Autodesk Fusion 360 part; units mm, degrees
(part 2 of 4)
  line L1019 (-48.5, -47.866) -> (-48, -48.7321)
  line L1020 (-40.5, -47.866) -> (-41, -47)
  line L1021 (-48.5, -41.866) -> (-48, -42.7321)
  line L1022 (-35, -36.7321) -> (-34.5, -35.866)
  line L1023 (-46.5, -41.866) -> (-47, -41)
  line L1024 (-39, -36.7321) -> (-38, -36.7321)
  line L1025 (-45, -42.7321) -> (-44, -42.7321)
  line L1026 (-47, -44) -> (-48, -44)
  line L1027 (-44, -47) -> (-45, -47)
  line L1028 (-48, -48.7321) -> (-47, -48.7321)
  line L1029 (-48, -44) -> (-48.5, -44.866)
  line L1030 (-35, -38) -> (-36, -38)
  line L1031 (-48, -41) -> (-48.5, -41.866)
  line L1032 (-45, -47) -> (-45.5, -47.866)
  line L1033 (-44, -41) -> (-45, -41)
  line L1034 (-38, -38) -> (-39, -38)
  line L1035 (-39, -39.7321) -> (-38, -39.7321)
  line L1036 (-45, -48.7321) -> (-44, -48.7321)
  line L1037 (-45, -41) -> (-45.5, -41.866)
  line L1038 (-42.5, -56.866) -> (-42, -57.7321)
  line L1039 (-40.5, -56.866) -> (-41, -56)
  line L1040 (-44, -54.7321) -> (-43.5, -53.866)
  line L1041 (-42, -51.7321) -> (-41, -51.7321)
  line L1042 (-41, -51.7321) -> (-40.5, -50.866)
  line L1043 (-44, -57.7321) -> (-43.5, -56.866)
  line L1044 (-38, -48.7321) -> (-37.5, -47.866)
  line L1045 (-40.5, -50.866) -> (-41, -50)
  line L1046 (-42, -57.7321) -> (-41, -57.7321)
  line L1047 (-36, -47) -> (-36.5, -47.866)
  line L1048 (-39.5, -47.866) -> (-39, -48.7321)
  line L1049 (-40.5, -53.866) -> (-41, -53)
  line L1050 (-39, -48.7321) -> (-38, -48.7321)
  line L1051 (-42.5, -53.866) -> (-42, -54.7321)
  line L1052 (-41, -57.7321) -> (-40.5, -56.866)
  line L1053 (-41, -50) -> (-42, -50)
  line L1054 (-45.5, -47.866) -> (-45, -48.7321)
  line L1055 (-42, -53) -> (-42.5, -53.866)
  line L1056 (-44, -51.7321) -> (-43.5, -50.866)
  line L1057 (-42, -50) -> (-42.5, -50.866)
  line L1058 (-36.5, -35.866) -> (-36, -36.7321)
  line L1059 (-45.5, -41.866) -> (-45, -42.7321)
  line L1060 (-42, -54.7321) -> (-41, -54.7321)
  line L1061 (-35, -39.7321) -> (-34.5, -38.866)
  line L1062 (-47, -42.7321) -> (-46.5, -41.866)
  line L1063 (-43.5, -53.866) -> (-44, -53)
  line L1064 (-38, -39.7321) -> (-37.5, -38.866)
  line L1065 (-42.5, -50.866) -> (-42, -51.7321)
  line L1066 (-43.5, -50.866) -> (-44, -50)
  line L1067 (-37.5, -38.866) -> (-38, -38)
  line L1068 (-36, -36.7321) -> (-35, -36.7321)
  line L1069 (-36, -39.7321) -> (-35, -39.7321)
  line L1070 (-45.5, -44.866) -> (-45, -45.7321)
  line L1071 (-38, -35) -> (-39, -35)
  line L1072 (-39.5, -38.866) -> (-39, -39.7321)
  line L1073 (-41, -54.7321) -> (-40.5, -53.866)
  line L1074 (-43.5, -56.866) -> (-44, -56)
  line L1075 (-42, -56) -> (-42.5, -56.866)
  line L1076 (-39.5, -35.866) -> (-39, -36.7321)
  line L1077 (-35, -35) -> (-36, -35)
  line L1078 (-41, -56) -> (-42, -56)
  line L1079 (-48, -47) -> (-48.5, -47.866)
  line L1080 (-39, -38) -> (-39.5, -38.866)
  line L1081 (-34.5, -38.866) -> (-35, -38)
  line L1082 (-41, -53) -> (-42, -53)
  line L1083 (-47, -48.7321) -> (-46.5, -47.866)
  line L1084 (-36, -35) -> (-36.5, -35.866)
  line L1085 (-46.5, -47.866) -> (-47, -47)
  line L1086 (-38, -36.7321) -> (-37.5, -35.866)
  line L1087 (-36, -38) -> (-36.5, -38.866)
  line L1088 (-36.5, -38.866) -> (-36, -39.7321)
  line L1089 (-48, -42.7321) -> (-47, -42.7321)
  line L1090 (-46.5, -44.866) -> (-47, -44)
  line L1091 (-34.5, -35.866) -> (-35, -35)
  line L1092 (-59, -54.7321) -> (-58.5, -53.866)
  line L1093 (-57, -47) -> (-57.5, -47.866)
  line L1094 (-60, -51.7321) -> (-59, -51.7321)
  line L1095 (-56, -47) -> (-57, -47)
  line L1096 (-60, -57.7321) -> (-59, -57.7321)
  line L1097 (-58.5, -56.866) -> (-59, -56)
  line L1098 (-53, -54.7321) -> (-52.5, -53.866)
  line L1099 (-52.5, -50.866) -> (-53, -50)
  line L1100 (-51, -56) -> (-51.5, -56.866)
  line L1101 (-50, -50) -> (-51, -50)
  line L1102 (-63, -54.7321) -> (-62, -54.7321)
  line L1103 (-59, -51.7321) -> (-58.5, -50.866)
  line L1104 (-53, -57.7321) -> (-52.5, -56.866)
  line L1105 (-50, -53) -> (-51, -53)
  line L1106 (-60, -54.7321) -> (-59, -54.7321)
  line L1107 (-54, -47) -> (-54.5, -47.866)
  line L1108 (-63.5, -56.866) -> (-63, -57.7321)
  line L1109 (-55.5, -47.866) -> (-56, -47)
  line L1110 (-57, -48.7321) -> (-56, -48.7321)
  line L1111 (-54.5, -44.866) -> (-54, -45.7321)
  line L1112 (-63, -53) -> (-63.5, -53.866)
  line L1113 (-62, -54.7321) -> (-61.5, -53.866)
  line L1114 (-51, -57.7321) -> (-50, -57.7321)
  line L1115 (-57, -41) -> (-57.5, -41.866)
  line L1116 (-60.5, -53.866) -> (-60, -54.7321)
  line L1117 (-57.5, -41.866) -> (-57, -42.7321)
  line L1118 (-63.5, -50.866) -> (-63, -51.7321)
  line L1119 (-60, -53) -> (-60.5, -53.866)
  line L1120 (-59, -50) -> (-60, -50)
  line L1121 (-56, -41) -> (-57, -41)
  line L1122 (-52.5, -53.866) -> (-53, -53)
  line L1123 (-63, -56) -> (-63.5, -56.866)
  line L1124 (-62, -56) -> (-63, -56)
  line L1125 (-60, -56) -> (-60.5, -56.866)
  line L1126 (-49.5, -50.866) -> (-50, -50)
  line L1127 (-62, -50) -> (-63, -50)
  line L1128 (-61.5, -53.866) -> (-62, -53)
  line L1129 (-60.5, -56.866) -> (-60, -57.7321)
  line L1130 (-62, -57.7321) -> (-61.5, -56.866)
  line L1131 (-59, -57.7321) -> (-58.5, -56.866)
  line L1132 (-61.5, -56.866) -> (-62, -56)
  line L1133 (-62, -51.7321) -> (-61.5, -50.866)
  line L1134 (-63, -50) -> (-63.5, -50.866)
  line L1135 (-58.5, -50.866) -> (-59, -50)
  line L1136 (-60, -50) -> (-60.5, -50.866)
  line L1137 (-57, -44) -> (-57.5, -44.866)
  line L1138 (-50, -51.7321) -> (-49.5, -50.866)
  line L1139 (-51, -47) -> (-51.5, -47.866)
  line L1140 (-51, -48.7321) -> (-50, -48.7321)
  line L1141 (-35, -54.7321) -> (-34.5, -53.866)
  line L1142 (-53, -48.7321) -> (-52.5, -47.866)
  line L1143 (-60.5, -38.866) -> (-60, -39.7321)
  line L1144 (-60, -36.7321) -> (-59, -36.7321)
  line L1145 (-38, -54.7321) -> (-37.5, -53.866)
  line L1146 (-52.5, -41.866) -> (-53, -41)
  line L1147 (-36.5, -53.866) -> (-36, -54.7321)
  line L1148 (-62, -38) -> (-63, -38)
  line L1149 (-58.5, -35.866) -> (-59, -35)
  line L1150 (-39, -53) -> (-39.5, -53.866)
  line L1151 (-51, -42.7321) -> (-50, -42.7321)
  line L1152 (-52.5, -47.866) -> (-53, -47)
  line L1153 (-53, -45.7321) -> (-52.5, -44.866)
  line L1154 (-60, -35) -> (-60.5, -35.866)
  line L1155 (-38, -50) -> (-39, -50)
  line L1156 (-50, -42.7321) -> (-49.5, -41.866)
  line L1157 (-63, -39.7321) -> (-62, -39.7321)
  line L1158 (-59, -35) -> (-60, -35)
  line L1159 (-63.5, -35.866) -> (-63, -36.7321)
  line L1160 (-63, -38) -> (-63.5, -38.866)
  line L1161 (-61.5, -35.866) -> (-62, -35)
  line L1162 (-60, -39.7321) -> (-59, -39.7321)
  line L1163 (-60.5, -35.866) -> (-60, -36.7321)
  line L1164 (-62, -36.7321) -> (-61.5, -35.866)
  line L1165 (-62, -39.7321) -> (-61.5, -38.866)
  line L1166 (-61.5, -38.866) -> (-62, -38)
  line L1167 (-51, -41) -> (-51.5, -41.866)
  line L1168 (-36, -56) -> (-36.5, -56.866)
  line L1169 (-51.5, -44.866) -> (-51, -45.7321)
  line L1170 (-36, -57.7321) -> (-35, -57.7321)
  line L1171 (-36, -53) -> (-36.5, -53.866)
  line L1172 (-34.5, -50.866) -> (-35, -50)
  line L1173 (-49.5, -41.866) -> (-50, -41)
  line L1174 (-35, -57.7321) -> (-34.5, -56.866)
  line L1175 (-37.5, -53.866) -> (-38, -53)
  line L1176 (-34.5, -56.866) -> (-35, -56)
  line L1177 (-37.5, -50.866) -> (-38, -50)
  line L1178 (-39, -54.7321) -> (-38, -54.7321)
  line L1179 (-38, -51.7321) -> (-37.5, -50.866)
  line L1180 (-36, -51.7321) -> (-35, -51.7321)
  line L1181 (-39.5, -53.866) -> (-39, -54.7321)
  line L1182 (-51.5, -41.866) -> (-51, -42.7321)
  line L1183 (-39.5, -56.866) -> (-39, -57.7321)
  line L1184 (-49.5, -44.866) -> (-50, -44)
  line L1185 (-50, -45.7321) -> (-49.5, -44.866)
  line L1186 (-57, -39.7321) -> (-56, -39.7321)
  line L1187 (-37.5, -56.866) -> (-38, -56)
  line L1188 (-38, -56) -> (-39, -56)
  line L1189 (-34.5, -53.866) -> (-35, -53)
  line L1190 (-36, -54.7321) -> (-35, -54.7321)
  line L1191 (-64.5, -56.866) -> (-65, -56)
  line L1192 (-64.5, -41.866) -> (-65, -41)
  line L1193 (-69.5, -50.866) -> (-69, -51.7321)
  line L1194 (-65, -42.7321) -> (-64.5, -41.866)
  line L1195 (-64.5, -44.866) -> (-65, -44)
  line L1196 (-66, -42.7321) -> (-65, -42.7321)
  line L1197 (-68, -50) -> (-69, -50)
  line L1198 (-66.5, -41.866) -> (-66, -42.7321)
  line L1199 (-69, -47) -> (-69.5, -47.866)
  line L1200 (-68, -51.7321) -> (-67.5, -50.866)
  line L1201 (-69, -56) -> (-69.5, -56.866)
  line L1202 (-66.5, -44.866) -> (-66, -45.7321)
  line L1203 (-68, -53) -> (-69, -53)
  line L1204 (-69, -51.7321) -> (-68, -51.7321)
  line L1205 (-67.5, -44.866) -> (-68, -44)
  line L1206 (-69, -53) -> (-69.5, -53.866)
  line L1207 (-66, -50) -> (-66.5, -50.866)
  line L1208 (-69, -57.7321) -> (-68, -57.7321)
  line L1209 (-66.5, -47.866) -> (-66, -48.7321)
  line L1210 (-68, -45.7321) -> (-67.5, -44.866)
  line L1211 (-66, -45.7321) -> (-65, -45.7321)
  line L1212 (-69.5, -56.866) -> (-69, -57.7321)
  line L1213 (-68, -42.7321) -> (-67.5, -41.866)
  line L1214 (-69, -42.7321) -> (-68, -42.7321)
  line L1215 (-69.5, -44.866) -> (-69, -45.7321)
  line L1216 (-66.5, -50.866) -> (-66, -51.7321)
  line L1217 (-69, -45.7321) -> (-68, -45.7321)
  line L1218 (-68, -48.7321) -> (-67.5, -47.866)
  line L1219 (-65, -44) -> (-66, -44)
  line L1220 (-11, -51.7321) -> (-10.5, -50.866)
  line L1221 (-21, -38) -> (-21.5, -38.866)
  line L1222 (-13.5, -38.866) -> (-14, -38)
  line L1223 (-16.5, -35.866) -> (-17, -35)
  line L1224 (-11, -50) -> (-12, -50)
  line L1225 (-12, -57.7321) -> (-11, -57.7321)
  line L1226 (-14, -35) -> (-15, -35)
  line L1227 (-24, -38) -> (-24.5, -38.866)
  line L1228 (-14, -53) -> (-15, -53)
  line L1229 (-18, -38) -> (-18.5, -38.866)
  line L1230 (-10.5, -35.866) -> (-11, -35)
  line L1231 (-17, -36.7321) -> (-16.5, -35.866)
  line L1232 (-11, -53) -> (-12, -53)
  line L1233 (-24.5, -35.866) -> (-24, -36.7321)
  line L1234 (-20, -35) -> (-21, -35)
  line L1235 (-12, -38) -> (-12.5, -38.866)
  line L1236 (-17, -39.7321) -> (-16.5, -38.866)
  line L1237 (-15.5, -50.866) -> (-15, -51.7321)
  line L1238 (-25.5, -35.866) -> (-26, -35)
  line L1239 (-18, -57.7321) -> (-17, -57.7321)
  line L1240 (-24, -36.7321) -> (-23, -36.7321)
  line L1241 (-12, -35) -> (-12.5, -35.866)
  line L1242 (-23, -39.7321) -> (-22.5, -38.866)
  line L1243 (-17, -38) -> (-18, -38)
  line L1244 (-21, -36.7321) -> (-20, -36.7321)
  line L1245 (-24, -39.7321) -> (-23, -39.7321)
  line L1246 (-12.5, -53.866) -> (-12, -54.7321)
  line L1247 (-18.5, -50.866) -> (-18, -51.7321)
  line L1248 (-14, -54.7321) -> (-13.5, -53.866)
  line L1249 (-14, -38) -> (-15, -38)
  line L1250 (-10.5, -38.866) -> (-11, -38)
  line L1251 (-24, -35) -> (-24.5, -35.866)
  line L1252 (-27, -35) -> (-27.5, -35.866)
  line L1253 (-22.5, -35.866) -> (-23, -35)
  line L1254 (-12, -36.7321) -> (-11, -36.7321)
  line L1255 (-22.5, -38.866) -> (-23, -38)
  line L1256 (-23, -38) -> (-24, -38)
  line L1257 (-14, -50) -> (-15, -50)
  line L1258 (-19.5, -35.866) -> (-20, -35)
  line L1259 (-11, -38) -> (-12, -38)
  line L1260 (-19.5, -38.866) -> (-20, -38)
  line L1261 (-11, -39.7321) -> (-10.5, -38.866)
  line L1262 (-12.5, -50.866) -> (-12, -51.7321)
  line L1263 (-15, -36.7321) -> (-14, -36.7321)
  line L1264 (-27.5, -38.866) -> (-27, -39.7321)
  line L1265 (-15, -35) -> (-15.5, -35.866)
  line L1266 (-12.5, -38.866) -> (-12, -39.7321)
  line L1267 (-27.5, -35.866) -> (-27, -36.7321)
  line L1268 (-14, -51.7321) -> (-13.5, -50.866)
  line L1269 (-21.5, -38.866) -> (-21, -39.7321)
  line L1270 (-11, -36.7321) -> (-10.5, -35.866)
  line L1271 (-27, -39.7321) -> (-26, -39.7321)
  line L1272 (-20, -38) -> (-21, -38)
  line L1273 (-11, -57.7321) -> (-10.5, -56.866)
  line L1274 (-12, -53) -> (-12.5, -53.866)
  line L1275 (-10.5, -50.866) -> (-11, -50)
  line L1276 (-12, -39.7321) -> (-11, -39.7321)
  line L1277 (-14, -57.7321) -> (-13.5, -56.866)
  line L1278 (-26, -39.7321) -> (-25.5, -38.866)
  line L1279 (-15, -39.7321) -> (-14, -39.7321)
  line L1280 (-15.5, -38.866) -> (-15, -39.7321)
  line L1281 (-18, -36.7321) -> (-17, -36.7321)
  line L1282 (-12.5, -56.866) -> (-12, -57.7321)
  line L1283 (-20, -36.7321) -> (-19.5, -35.866)
  line L1284 (-13.5, -56.866) -> (-14, -56)
  line L1285 (-24.5, -38.866) -> (-24, -39.7321)
  line L1286 (-18, -39.7321) -> (-17, -39.7321)
  line L1287 (-12, -54.7321) -> (-11, -54.7321)
  line L1288 (-10.5, -56.866) -> (-11, -56)
  line L1289 (-14, -36.7321) -> (-13.5, -35.866)
  line L1290 (-10.5, -53.866) -> (-11, -53)
  line L1291 (-21.5, -35.866) -> (-21, -36.7321)
  line L1292 (-12.5, -35.866) -> (-12, -36.7321)
  line L1293 (-21, -39.7321) -> (-20, -39.7321)
  line L1294 (-14, -39.7321) -> (-13.5, -38.866)
  line L1295 (-12, -50) -> (-12.5, -50.866)
  line L1296 (-12, -51.7321) -> (-11, -51.7321)
  line L1297 (-26, -36.7321) -> (-25.5, -35.866)
  line L1298 (-18, -35) -> (-18.5, -35.866)
  line L1299 (-27, -38) -> (-27.5, -38.866)
  line L1300 (-13.5, -35.866) -> (-14, -35)
  line L1301 (-23, -42.7321) -> (-22.5, -41.866)
  line L1302 (-22.5, -44.866) -> (-23, -44)
  line L1303 (-21, -45.7321) -> (-20, -45.7321)
  line L1304 (-20, -44) -> (-21, -44)
  line L1305 (-25.5, -38.866) -> (-26, -38)
  line L1306 (-26, -38) -> (-27, -38)
  line L1307 (-22.5, -47.866) -> (-23, -47)
  line L1308 (-17, -51.7321) -> (-16.5, -50.866)
  line L1309 (-17, -50) -> (-18, -50)
  line L1310 (-15, -53) -> (-15.5, -53.866)
  line L1311 (-16.5, -38.866) -> (-17, -38)
  line L1312 (-16.5, -53.866) -> (-17, -53)
  line L1313 (-14, -56) -> (-15, -56)
  line L1314 (-20, -39.7321) -> (-19.5, -38.866)
  line L1315 (-18, -50) -> (-18.5, -50.866)
  line L1316 (-21, -35) -> (-21.5, -35.866)
  line L1317 (-18.5, -38.866) -> (-18, -39.7321)
  line L1318 (-17, -56) -> (-18, -56)
  line L1319 (-20, -41) -> (-21, -41)
  line L1320 (-15, -50) -> (-15.5, -50.866)
  line L1321 (-15.5, -53.866) -> (-15, -54.7321)
  line L1322 (-17, -53) -> (-18, -53)
  line L1323 (-18.5, -53.866) -> (-18, -54.7321)
  line L1324 (-19.5, -41.866) -> (-20, -41)
  line L1325 (-15, -54.7321) -> (-14, -54.7321)
  line L1326 (-16.5, -50.866) -> (-17, -50)
  line L1327 (-22.5, -41.866) -> (-23, -41)
  line L1328 (-19.5, -47.866) -> (-20, -47)
  line L1329 (-18, -51.7321) -> (-17, -51.7321)
  line L1330 (-18, -53) -> (-18.5, -53.866)
  line L1331 (-18, -54.7321) -> (-17, -54.7321)
  line L1332 (-17, -57.7321) -> (-16.5, -56.866)
  line L1333 (-21, -42.7321) -> (-20, -42.7321)
  line L1334 (-20, -47) -> (-21, -47)
  line L1335 (-17, -54.7321) -> (-16.5, -53.866)
  line L1336 (-15, -51.7321) -> (-14, -51.7321)
  line L1337 (-23, -48.7321) -> (-22.5, -47.866)
  line L1338 (-15.5, -56.866) -> (-15, -57.7321)
  line L1339 (-21.5, -41.866) -> (-21, -42.7321)
  line L1340 (-20, -45.7321) -> (-19.5, -44.866)
  line L1341 (-15, -56) -> (-15.5, -56.866)
  line L1342 (-18, -56) -> (-18.5, -56.866)
  line L1343 (-15, -57.7321) -> (-14, -57.7321)
  line L1344 (-19.5, -44.866) -> (-20, -44)
  line L1345 (-29, -39.7321) -> (-28.5, -38.866)
  line L1346 (-16.5, -56.866) -> (-17, -56)
  line L1347 (-18.5, -56.866) -> (-18, -57.7321)
  line L1348 (-21, -41) -> (-21.5, -41.866)
  line L1349 (-23, -47) -> (-24, -47)
  line L1350 (-26, -41) -> (-27, -41)
  line L1351 (-32, -36.7321) -> (-31.5, -35.866)
  line L1352 (-21.5, -47.866) -> (-21, -48.7321)
  line L1353 (-24, -42.7321) -> (-23, -42.7321)
  line L1354 (-26, -42.7321) -> (-25.5, -41.866)
  line L1355 (-27, -42.7321) -> (-26, -42.7321)
  line L1356 (-29, -38) -> (-30, -38)
  line L1357 (-27, -48.7321) -> (-26, -48.7321)
  line L1358 (-33.5, -35.866) -> (-33, -36.7321)
  line L1359 (-24.5, -44.866) -> (-24, -45.7321)
  line L1360 (-21, -47) -> (-21.5, -47.866)
  line L1361 (-20, -48.7321) -> (-19.5, -47.866)
  line L1362 (-23, -44) -> (-24, -44)
  line L1363 (-27.5, -41.866) -> (-27, -42.7321)
  line L1364 (-24.5, -47.866) -> (-24, -48.7321)
  line L1365 (-31.5, -35.866) -> (-32, -35)
  line L1366 (-23, -45.7321) -> (-22.5, -44.866)
  line L1367 (-21.5, -44.866) -> (-21, -45.7321)
  line L1368 (-24, -45.7321) -> (-23, -45.7321)
  line L1369 (-28.5, -38.866) -> (-29, -38)
  line L1370 (-33.5, -38.866) -> (-33, -39.7321)
  line L1371 (-21, -48.7321) -> (-20, -48.7321)
  line L1372 (-21, -44) -> (-21.5, -44.866)
  line L1373 (-20, -42.7321) -> (-19.5, -41.866)
  line L1374 (-26, -45.7321) -> (-25.5, -44.866)
  line L1375 (-29, -36.7321) -> (-28.5, -35.866)
  line L1376 (-27.5, -44.866) -> (-27, -45.7321)
  line L1377 (-29, -51.7321) -> (-28.5, -50.866)
  line L1378 (-44, -35) -> (-45, -35)
  line L1379 (-28.5, -50.866) -> (-29, -50)
  line L1380 (-41, -39.7321) -> (-40.5, -38.866)
  line L1381 (-31.5, -56.866) -> (-32, -56)
  line L1382 (-45, -36.7321) -> (-44, -36.7321)
  line L1383 (-43.5, -35.866) -> (-44, -35)
  line L1384 (-44, -36.7321) -> (-43.5, -35.866)
  line L1385 (-48, -39.7321) -> (-47, -39.7321)
  line L1386 (-32, -54.7321) -> (-31.5, -53.866)
  line L1387 (-43.5, -38.866) -> (-44, -38)
  line L1388 (-42, -35) -> (-42.5, -35.866)
  line L1389 (-42.5, -35.866) -> (-42, -36.7321)
  line L1390 (-28.5, -56.866) -> (-29, -56)
  line L1391 (-31.5, -53.866) -> (-32, -53)
  line L1392 (-42.5, -38.866) -> (-42, -39.7321)
  line L1393 (-33, -53) -> (-33.5, -53.866)
  line L1394 (-29, -54.7321) -> (-28.5, -53.866)
  line L1395 (-33.5, -53.866) -> (-33, -54.7321)
  line L1396 (-28.5, -53.866) -> (-29, -53)
  line L1397 (-45.5, -38.866) -> (-45, -39.7321)
  line L1398 (-47, -39.7321) -> (-46.5, -38.866)
  line L1399 (-40.5, -41.866) -> (-41, -41)
  line L1400 (-30.5, -50.866) -> (-30, -51.7321)
  line L1401 (-42, -38) -> (-42.5, -38.866)
  line L1402 (-29, -56) -> (-30, -56)
  line L1403 (-33, -50) -> (-33.5, -50.866)
  line L1404 (-33, -54.7321) -> (-32, -54.7321)
  line L1405 (-33, -57.7321) -> (-32, -57.7321)
  line L1406 (-48.5, -38.866) -> (-48, -39.7321)
  line L1407 (-40.5, -38.866) -> (-41, -38)
  line L1408 (-45, -38) -> (-45.5, -38.866)
  line L1409 (-44, -38) -> (-45, -38)
  line L1410 (-32, -56) -> (-33, -56)
  line L1411 (-32, -51.7321) -> (-31.5, -50.866)
  line L1412 (-41, -38) -> (-42, -38)
  line L1413 (-45, -35) -> (-45.5, -35.866)
  line L1414 (-30, -50) -> (-30.5, -50.866)
  line L1415 (-41, -35) -> (-42, -35)
  line L1416 (-32, -53) -> (-33, -53)
  line L1417 (-51.5, -35.866) -> (-51, -36.7321)
  line L1418 (-57.5, -38.866) -> (-57, -39.7321)
  line L1419 (-53, -36.7321) -> (-52.5, -35.866)
  line L1420 (-51.5, -38.866) -> (-51, -39.7321)
  line L1421 (-39, -51.7321) -> (-38, -51.7321)
  line L1422 (-54, -35) -> (-54.5, -35.866)
  line L1423 (-56, -35) -> (-57, -35)
  line L1424 (-54, -39.7321) -> (-53, -39.7321)
  line L1425 (-53, -38) -> (-54, -38)
  line L1426 (-39, -50) -> (-39.5, -50.866)
  line L1427 (-57, -38) -> (-57.5, -38.866)
  line L1428 (-35, -51.7321) -> (-34.5, -50.866)
  line L1429 (-50, -39.7321) -> (-49.5, -38.866)
  line L1430 (-50, -38) -> (-51, -38)
  line L1431 (-21, -57.7321) -> (-20, -57.7321)
  line L1432 (-30, -39.7321) -> (-29, -39.7321)
  line L1433 (-21.5, -53.866) -> (-21, -54.7321)
  line L1434 (-32, -39.7321) -> (-31.5, -38.866)
  line L1435 (-24, -41) -> (-24.5, -41.866)
  line L1436 (-33, -36.7321) -> (-32, -36.7321)
  line L1437 (-27, -47) -> (-27.5, -47.866)
  line L1438 (-23, -41) -> (-24, -41)
  line L1439 (-33, -39.7321) -> (-32, -39.7321)
  line L1440 (-30, -38) -> (-30.5, -38.866)
  line L1441 (-25.5, -44.866) -> (-26, -44)
  line L1442 (-23, -51.7321) -> (-22.5, -50.866)
  line L1443 (-30, -36.7321) -> (-29, -36.7321)
  line L1444 (-25.5, -41.866) -> (-26, -41)
  line L1445 (-32, -38) -> (-33, -38)
  line L1446 (-21, -56) -> (-21.5, -56.866)
  line L1447 (-32, -35) -> (-33, -35)
  line L1448 (-29, -35) -> (-30, -35)
  line L1449 (-21, -51.7321) -> (-20, -51.7321)
  line L1450 (-24, -47) -> (-24.5, -47.866)
  line L1451 (-24, -44) -> (-24.5, -44.866)
  line L1452 (-30.5, -35.866) -> (-30, -36.7321)
  line L1453 (-33, -38) -> (-33.5, -38.866)
  line L1454 (-31.5, -38.866) -> (-32, -38)
  line L1455 (-24.5, -41.866) -> (-24, -42.7321)
  line L1456 (-27, -45.7321) -> (-26, -45.7321)
  line L1457 (-30, -35) -> (-30.5, -35.866)
  line L1458 (-27.5, -47.866) -> (-27, -48.7321)
  line L1459 (-28.5, -35.866) -> (-29, -35)
  line L1460 (-26, -48.7321) -> (-25.5, -47.866)
  line L1461 (-25.5, -47.866) -> (-26, -47)
  line L1462 (-24, -48.7321) -> (-23, -48.7321)
  line L1463 (-30.5, -38.866) -> (-30, -39.7321)
  line L1464 (-27, -44) -> (-27.5, -44.866)
  line L1465 (-26, -44) -> (-27, -44)
  line L1466 (-27, -41) -> (-27.5, -41.866)
  line L1467 (-33, -35) -> (-33.5, -35.866)
  line L1468 (-26, -47) -> (-27, -47)
  line L1469 (-32, -47) -> (-33, -47)
  line L1470 (-29, -47) -> (-30, -47)
  line L1471 (-33.5, -41.866) -> (-33, -42.7321)
  line L1472 (-30.5, -41.866) -> (-30, -42.7321)
  line L1473 (-22.5, -53.866) -> (-23, -53)
  line L1474 (-21, -50) -> (-21.5, -50.866)
  line L1475 (-30, -47) -> (-30.5, -47.866)
  line L1476 (-21.5, -50.866) -> (-21, -51.7321)
  line L1477 (-21.5, -56.866) -> (-21, -57.7321)
  line L1478 (-20, -50) -> (-21, -50)
  line L1479 (-20, -53) -> (-21, -53)
  line L1480 (-33, -44) -> (-33.5, -44.866)
  line L1481 (-31.5, -41.866) -> (-32, -41)
  line L1482 (-31.5, -47.866) -> (-32, -47)
  line L1483 (-20, -51.7321) -> (-19.5, -50.866)
  line L1484 (-20, -56) -> (-21, -56)
  line L1485 (-23, -57.7321) -> (-22.5, -56.866)
  line L1486 (-30.5, -47.866) -> (-30, -48.7321)
  line L1487 (-33, -45.7321) -> (-32, -45.7321)
  line L1488 (-21, -54.7321) -> (-20, -54.7321)
  line L1489 (-23, -54.7321) -> (-22.5, -53.866)
  line L1490 (-19.5, -53.866) -> (-20, -53)
  line L1491 (-30, -42.7321) -> (-29, -42.7321)
  line L1492 (-29, -45.7321) -> (-28.5, -44.866)
  line L1493 (-20, -57.7321) -> (-19.5, -56.866)
  line L1494 (-19.5, -50.866) -> (-20, -50)
  line L1495 (-28.5, -47.866) -> (-29, -47)
  line L1496 (-22.5, -50.866) -> (-23, -50)
  line L1497 (-21, -53) -> (-21.5, -53.866)
  line L1498 (-19.5, -56.866) -> (-20, -56)
  line L1499 (-22.5, -56.866) -> (-23, -56)
  line L1500 (-20, -54.7321) -> (-19.5, -53.866)
  line L1501 (-13.5, -41.866) -> (-14, -41)
  line L1502 (-15, -38) -> (-15.5, -38.866)
  line L1503 (-16.5, -44.866) -> (-17, -44)
  line L1504 (-13.5, -50.866) -> (-14, -50)
  line L1505 (-13.5, -44.866) -> (-14, -44)
  line L1506 (-11, -54.7321) -> (-10.5, -53.866)
  line L1507 (-12, -44) -> (-12.5, -44.866)
  line L1508 (-18, -41) -> (-18.5, -41.866)
  line L1509 (-18.5, -35.866) -> (-18, -36.7321)
  line L1510 (-15, -48.7321) -> (-14, -48.7321)
  line L1511 (-10.5, -41.866) -> (-11, -41)
  line L1512 (-11, -42.7321) -> (-10.5, -41.866)
  line L1513 (-12.5, -41.866) -> (-12, -42.7321)
  line L1514 (-11, -47) -> (-12, -47)
  line L1515 (-13.5, -47.866) -> (-14, -47)
  line L1516 (-11, -56) -> (-12, -56)
  line L1517 (-15, -42.7321) -> (-14, -42.7321)
  line L1518 (-17, -48.7321) -> (-16.5, -47.866)
  line L1519 (-16.5, -47.866) -> (-17, -47)
  line L1520 (-17, -45.7321) -> (-16.5, -44.866)
  line L1521 (-11, -48.7321) -> (-10.5, -47.866)
  line L1522 (-27, -36.7321) -> (-26, -36.7321)
  line L1523 (-14, -47) -> (-15, -47)
  line L1524 (-14, -42.7321) -> (-13.5, -41.866)
  line L1525 (-14, -41) -> (-15, -41)
  line L1526 (-11, -35) -> (-12, -35)
  line L1527 (-17, -35) -> (-18, -35)
  line L1528 (-18.5, -47.866) -> (-18, -48.7321)
  line L1529 (-15.5, -44.866) -> (-15, -45.7321)
  line L1530 (-10.5, -44.866) -> (-11, -44)
  line L1531 (-26, -35) -> (-27, -35)
  line L1532 (-13.5, -53.866) -> (-14, -53)
  line L1533 (-17, -41) -> (-18, -41)
  line L1534 (-15.5, -35.866) -> (-15, -36.7321)
  line L1535 (-12, -41) -> (-12.5, -41.866)
  line L1536 (-15, -45.7321) -> (-14, -45.7321)
  line L1537 (-11, -44) -> (-12, -44)
  line L1538 (-14, -45.7321) -> (-13.5, -44.866)
  line L1539 (-23, -36.7321) -> (-22.5, -35.866)
  line L1540 (-23, -35) -> (-24, -35)
  line L1541 (-12, -56) -> (-12.5, -56.866)
  line L1542 (-17, -44) -> (-18, -44)
  line L1543 (-12, -47) -> (-12.5, -47.866)
  line L1544 (-11, -45.7321) -> (-10.5, -44.866)
  line L1545 (-11, -41) -> (-12, -41)
  line L1546 (-18.5, -41.866) -> (-18, -42.7321)
  line L1547 (-12, -45.7321) -> (-11, -45.7321)
  line L1548 (-12, -48.7321) -> (-11, -48.7321)
  line L1549 (-15, -41) -> (-15.5, -41.866)
  line L1550 (-10.5, -47.866) -> (-11, -47)
  line L1551 (-12.5, -44.866) -> (-12, -45.7321)
  line L1552 (-16.5, -41.866) -> (-17, -41)
  line L1553 (-12.5, -47.866) -> (-12, -48.7321)
  line L1554 (-15.5, -41.866) -> (-15, -42.7321)
  line L1555 (-14, -48.7321) -> (-13.5, -47.866)
  line L1556 (-18, -48.7321) -> (-17, -48.7321)
  line L1557 (-18.5, -44.866) -> (-18, -45.7321)
  line L1558 (-15, -44) -> (-15.5, -44.866)
  line L1559 (-17, -47) -> (-18, -47)
  line L1560 (-15, -47) -> (-15.5, -47.866)
  line L1561 (-14, -44) -> (-15, -44)
  line L1562 (-18, -44) -> (-18.5, -44.866)
  line L1563 (-15.5, -47.866) -> (-15, -48.7321)
  line L1564 (-18, -42.7321) -> (-17, -42.7321)
  line L1565 (-17, -42.7321) -> (-16.5, -41.866)
  line L1566 (-12, -42.7321) -> (-11, -42.7321)
  line L1567 (-18, -45.7321) -> (-17, -45.7321)
  line L1568 (-18, -47) -> (-18.5, -47.866)
  line L1569 (-52.5, -44.866) -> (-53, -44)
  line L1570 (-50, -47) -> (-51, -47)
  line L1571 (-61.5, -47.866) -> (-62, -47)
  line L1572 (-60, -42.7321) -> (-59, -42.7321)
  line L1573 (-63, -35) -> (-63.5, -35.866)
  line L1574 (-50, -41) -> (-51, -41)
  line L1575 (-59, -42.7321) -> (-58.5, -41.866)
  line L1576 (-60.5, -44.866) -> (-60, -45.7321)
  line L1577 (-59, -41) -> (-60, -41)
  line L1578 (-60, -48.7321) -> (-59, -48.7321)
  line L1579 (-58.5, -41.866) -> (-59, -41)
  line L1580 (-60, -45.7321) -> (-59, -45.7321)
  line L1581 (-60, -47) -> (-60.5, -47.866)
  line L1582 (-62, -42.7321) -> (-61.5, -41.866)
  line L1583 (-63.5, -41.866) -> (-63, -42.7321)
  line L1584 (-59, -48.7321) -> (-58.5, -47.866)
  line L1585 (-63, -48.7321) -> (-62, -48.7321)
  line L1586 (-59, -39.7321) -> (-58.5, -38.866)
  line L1587 (-63.5, -47.866) -> (-63, -48.7321)
  line L1588 (-59, -45.7321) -> (-58.5, -44.866)
  line L1589 (-58.5, -47.866) -> (-59, -47)
  line L1590 (-51.5, -47.866) -> (-51, -48.7321)
  line L1591 (-62, -47) -> (-63, -47)
  line L1592 (-59, -47) -> (-60, -47)
  line L1593 (-50, -44) -> (-51, -44)
  line L1594 (-61.5, -44.866) -> (-62, -44)
  line L1595 (-51, -45.7321) -> (-50, -45.7321)
  line L1596 (-58.5, -44.866) -> (-59, -44)
  line L1597 (-63, -47) -> (-63.5, -47.866)
  line L1598 (-62, -48.7321) -> (-61.5, -47.866)
  line L1599 (-61.5, -41.866) -> (-62, -41)
  line L1600 (-59, -38) -> (-60, -38)
  line L1601 (-62, -45.7321) -> (-61.5, -44.866)
  line L1602 (-51, -44) -> (-51.5, -44.866)
  line L1603 (-60, -38) -> (-60.5, -38.866)
  line L1604 (-63, -41) -> (-63.5, -41.866)
  line L1605 (-62, -41) -> (-63, -41)
  line L1606 (-63.5, -38.866) -> (-63, -39.7321)
  line L1607 (-49.5, -47.866) -> (-50, -47)
  line L1608 (-53, -42.7321) -> (-52.5, -41.866)
  line L1609 (-50, -48.7321) -> (-49.5, -47.866)
  line L1610 (-62, -35) -> (-63, -35)
  line L1611 (-59, -36.7321) -> (-58.5, -35.866)
  line L1612 (-63, -36.7321) -> (-62, -36.7321)
  line L1613 (-58.5, -38.866) -> (-59, -38)
  line L1614 (-63, -42.7321) -> (-62, -42.7321)
  line L1615 (-61.5, -50.866) -> (-62, -50)
  line L1616 (-54.5, -47.866) -> (-54, -48.7321)
  line L1617 (-63.5, -44.866) -> (-63, -45.7321)
  line L1618 (-56, -45.7321) -> (-55.5, -44.866)
  line L1619 (-60, -44) -> (-60.5, -44.866)
  line L1620 (-63, -44) -> (-63.5, -44.866)
  line L1621 (-54, -42.7321) -> (-53, -42.7321)
  line L1622 (-57, -42.7321) -> (-56, -42.7321)
  line L1623 (-62, -53) -> (-63, -53)
  line L1624 (-58.5, -53.866) -> (-59, -53)
  line L1625 (-59, -53) -> (-60, -53)
  line L1626 (-63, -51.7321) -> (-62, -51.7321)
  line L1627 (-54, -44) -> (-54.5, -44.866)
  line L1628 (-55.5, -41.866) -> (-56, -41)
  line L1629 (-56, -48.7321) -> (-55.5, -47.866)
  line L1630 (-57, -45.7321) -> (-56, -45.7321)
  line L1631 (-60.5, -41.866) -> (-60, -42.7321)
  line L1632 (-62, -44) -> (-63, -44)
  line L1633 (-54, -41) -> (-54.5, -41.866)
  line L1634 (-63, -57.7321) -> (-62, -57.7321)
  line L1635 (-54.5, -41.866) -> (-54, -42.7321)
  line L1636 (-59, -56) -> (-60, -56)
  line L1637 (-53, -41) -> (-54, -41)
  line L1638 (-56, -42.7321) -> (-55.5, -41.866)
  line L1639 (-59, -44) -> (-60, -44)
  line L1640 (-60.5, -47.866) -> (-60, -48.7321)
  line L1641 (-54, -45.7321) -> (-53, -45.7321)
  line L1642 (-57.5, -44.866) -> (-57, -45.7321)
  line L1643 (-55.5, -44.866) -> (-56, -44)
  line L1644 (-56, -44) -> (-57, -44)
  line L1645 (-63, -45.7321) -> (-62, -45.7321)
  line L1646 (-54, -48.7321) -> (-53, -48.7321)
  line L1647 (-53, -44) -> (-54, -44)
  line L1648 (-53, -47) -> (-54, -47)
  line L1649 (-57.5, -47.866) -> (-57, -48.7321)
  line L1650 (-60, -41) -> (-60.5, -41.866)
  line L1651 (-53, -51.7321) -> (-52.5, -50.866)
  line L1652 (-64.5, -35.866) -> (-65, -35)
  line L1653 (-66, -35) -> (-66.5, -35.866)
  line L1654 (-57, -57.7321) -> (-56, -57.7321)
  line L1655 (-60.5, -50.866) -> (-60, -51.7321)
  line L1656 (-66, -39.7321) -> (-65, -39.7321)
  line L1657 (-50, -56) -> (-51, -56)
  line L1658 (-57, -50) -> (-57.5, -50.866)
  line L1659 (-51.5, -56.866) -> (-51, -57.7321)
  line L1660 (-51.5, -50.866) -> (-51, -51.7321)
  line L1661 (-49.5, -56.866) -> (-50, -56)
  line L1662 (-69, -36.7321) -> (-68, -36.7321)
  line L1663 (-56, -54.7321) -> (-55.5, -53.866)
  line L1664 (-51, -50) -> (-51.5, -50.866)
  line L1665 (-51, -53) -> (-51.5, -53.866)
  line L1666 (-51.5, -53.866) -> (-51, -54.7321)
  line L1667 (-49.5, -53.866) -> (-50, -53)
  line L1668 (-65, -39.7321) -> (-64.5, -38.866)
  line L1669 (-69, -39.7321) -> (-68, -39.7321)
  line L1670 (-68, -39.7321) -> (-67.5, -38.866)
  line L1671 (-69.5, -38.866) -> (-69, -39.7321)
  line L1672 (-53, -56) -> (-54, -56)
  line L1673 (-55.5, -50.866) -> (-56, -50)
  line L1674 (-65, -38) -> (-66, -38)
  line L1675 (-54.5, -50.866) -> (-54, -51.7321)
  line L1676 (-57, -56) -> (-57.5, -56.866)
  line L1677 (-54, -53) -> (-54.5, -53.866)
  line L1678 (-54.5, -56.866) -> (-54, -57.7321)
  line L1679 (-68, -35) -> (-69, -35)
  line L1680 (-53, -50) -> (-54, -50)
  line L1681 (-64.5, -38.866) -> (-65, -38)
  line L1682 (-69, -38) -> (-69.5, -38.866)
  line L1683 (-65, -36.7321) -> (-64.5, -35.866)
  line L1684 (-65, -35) -> (-66, -35)
  line L1685 (-66, -38) -> (-66.5, -38.866)
  line L1686 (-68, -38) -> (-69, -38)
  line L1687 (-69.5, -35.866) -> (-69, -36.7321)
  line L1688 (-69, -35) -> (-69.5, -35.866)
  line L1689 (-51, -51.7321) -> (-50, -51.7321)
  line L1690 (-50, -57.7321) -> (-49.5, -56.866)
  line L1691 (-50, -54.7321) -> (-49.5, -53.866)
  line L1692 (-52.5, -56.866) -> (-53, -56)
  line L1693 (-51, -54.7321) -> (-50, -54.7321)
  line L1694 (-63.5, -53.866) -> (-63, -54.7321)
  line L1695 (-36.5, -56.866) -> (-36, -57.7321)
  line L1696 (-39, -57.7321) -> (-38, -57.7321)
  line L1697 (-38, -53) -> (-39, -53)
  line L1698 (-57, -35) -> (-57.5, -35.866)
  line L1699 (-35, -50) -> (-36, -50)
  line L1700 (-52.5, -35.866) -> (-53, -35)
  line L1701 (-57.5, -35.866) -> (-57, -36.7321)
  line L1702 (-52.5, -38.866) -> (-53, -38)
  line L1703 (-38, -57.7321) -> (-37.5, -56.866)
  line L1704 (-35, -53) -> (-36, -53)
  line L1705 (-51, -36.7321) -> (-50, -36.7321)
  line L1706 (-56, -39.7321) -> (-55.5, -38.866)
  line L1707 (-39.5, -50.866) -> (-39, -51.7321)
  line L1708 (-54, -38) -> (-54.5, -38.866)
  line L1709 (-53, -35) -> (-54, -35)
  line L1710 (-50, -35) -> (-51, -35)
  line L1711 (-54, -36.7321) -> (-53, -36.7321)
  line L1712 (-47, -57.7321) -> (-46.5, -56.866)
  line L1713 (-39, -42.7321) -> (-38, -42.7321)
  line L1714 (-45, -51.7321) -> (-44, -51.7321)
  line L1715 (-38, -42.7321) -> (-37.5, -41.866)
  line L1716 (-51, -35) -> (-51.5, -35.866)
  line L1717 (-55.5, -38.866) -> (-56, -38)
  line L1718 (-49.5, -38.866) -> (-50, -38)
  line L1719 (-36.5, -44.866) -> (-36, -45.7321)
  line L1720 (-56, -36.7321) -> (-55.5, -35.866)
  line L1721 (-36, -42.7321) -> (-35, -42.7321)
  line L1722 (-51, -38) -> (-51.5, -38.866)
  line L1723 (-35, -42.7321) -> (-34.5, -41.866)
  line L1724 (-45.5, -50.866) -> (-45, -51.7321)
  line L1725 (-34.5, -44.866) -> (-35, -44)
  line L1726 (-55.5, -35.866) -> (-56, -35)
  line L1727 (-54.5, -38.866) -> (-54, -39.7321)
  line L1728 (-53, -39.7321) -> (-52.5, -38.866)
  line L1729 (-54.5, -35.866) -> (-54, -36.7321)
  line L1730 (-36.5, -41.866) -> (-36, -42.7321)
  line L1731 (-39, -47) -> (-39.5, -47.866)
  line L1732 (-45.5, -53.866) -> (-45, -54.7321)
  line L1733 (-50, -36.7321) -> (-49.5, -35.866)
  line L1734 (-47, -54.7321) -> (-46.5, -53.866)
  line L1735 (-39, -41) -> (-39.5, -41.866)
  line L1736 (-39.5, -44.866) -> (-39, -45.7321)
  line L1737 (-37.5, -44.866) -> (-38, -44)
  line L1738 (-38, -44) -> (-39, -44)
  line L1739 (-57, -36.7321) -> (-56, -36.7321)
  line L1740 (-36, -48.7321) -> (-35, -48.7321)
  line L1741 (-49.5, -35.866) -> (-50, -35)
  line L1742 (-66, -57.7321) -> (-65, -57.7321)
  line L1743 (-66, -51.7321) -> (-65, -51.7321)
  line L1744 (-64.5, -53.866) -> (-65, -53)
  line L1745 (-66, -54.7321) -> (-65, -54.7321)
  line L1746 (-65, -54.7321) -> (-64.5, -53.866)
  line L1747 (-69, -50) -> (-69.5, -50.866)
  line L1748 (-64.5, -50.866) -> (-65, -50)
  line L1749 (-68, -57.7321) -> (-67.5, -56.866)
  line L1750 (-65, -53) -> (-66, -53)
  line L1751 (-65, -56) -> (-66, -56)
  line L1752 (-65, -50) -> (-66, -50)
  line L1753 (-69.5, -53.866) -> (-69, -54.7321)
  line L1754 (-65, -51.7321) -> (-64.5, -50.866)
  line L1755 (-68, -56) -> (-69, -56)
  line L1756 (-65, -57.7321) -> (-64.5, -56.866)
  line L1757 (-67.5, -53.866) -> (-68, -53)
  line L1758 (-69, -54.7321) -> (-68, -54.7321)
  line L1759 (-66, -53) -> (-66.5, -53.866)
  line L1760 (-67.5, -50.866) -> (-68, -50)
  line L1761 (-67.5, -56.866) -> (-68, -56)
  line L1762 (-66.5, -56.866) -> (-66, -57.7321)
  line L1763 (-51, -39.7321) -> (-50, -39.7321)
  line L1764 (-35, -56) -> (-36, -56)
  line L1765 (-56, -38) -> (-57, -38)
  line L1766 (-36.5, -50.866) -> (-36, -51.7321)
  line L1767 (-39, -56) -> (-39.5, -56.866)
  line L1768 (-36, -50) -> (-36.5, -50.866)
  line L1769 (-31.5, -50.866) -> (-32, -50)
  line L1770 (-41, -42.7321) -> (-40.5, -41.866)
  line L1771 (-42, -41) -> (-42.5, -41.866)
  line L1772 (-40.5, -44.866) -> (-41, -44)
  line L1773 (-32, -50) -> (-33, -50)
  line L1774 (-33.5, -50.866) -> (-33, -51.7321)
  line L1775 (-42, -42.7321) -> (-41, -42.7321)
  line L1776 (-41, -47) -> (-42, -47)
  line L1777 (-42, -45.7321) -> (-41, -45.7321)
  line L1778 (-42, -48.7321) -> (-41, -48.7321)
  line L1779 (-33.5, -56.866) -> (-33, -57.7321)
  line L1780 (-44, -42.7321) -> (-43.5, -41.866)
  line L1781 (-43.5, -44.866) -> (-44, -44)
  line L1782 (-29, -53) -> (-30, -53)
  line L1783 (-29, -57.7321) -> (-28.5, -56.866)
  line L1784 (-41, -45.7321) -> (-40.5, -44.866)
  line L1785 (-33, -51.7321) -> (-32, -51.7321)
  line L1786 (-41, -41) -> (-42, -41)
  line L1787 (-43.5, -47.866) -> (-44, -47)
  line L1788 (-29, -50) -> (-30, -50)
  line L1789 (-42, -44) -> (-42.5, -44.866)
  line L1790 (-30, -54.7321) -> (-29, -54.7321)
  line L1791 (-30, -57.7321) -> (-29, -57.7321)
  line L1792 (-44, -45.7321) -> (-43.5, -44.866)
  line L1793 (-42, -47) -> (-42.5, -47.866)
  line L1794 (-30.5, -56.866) -> (-30, -57.7321)
  line L1795 (-44, -48.7321) -> (-43.5, -47.866)
  line L1796 (-30, -51.7321) -> (-29, -51.7321)
  line L1797 (-43.5, -41.866) -> (-44, -41)
  line L1798 (-41, -48.7321) -> (-40.5, -47.866)
  line L1799 (-42.5, -44.866) -> (-42, -45.7321)
  line L1800 (-30, -53) -> (-30.5, -53.866)
  line L1801 (-30.5, -53.866) -> (-30, -54.7321)
  line L1802 (-41, -44) -> (-42, -44)
  line L1803 (-30, -56) -> (-30.5, -56.866)
  line L1804 (-42.5, -47.866) -> (-42, -48.7321)
  line L1805 (-42.5, -41.866) -> (-42, -42.7321)
  line L1806 (-67.5, -38.866) -> (-68, -38)
  line L1807 (-68, -54.7321) -> (-67.5, -53.866)
  line L1808 (-66, -56) -> (-66.5, -56.866)
  line L1809 (-66.5, -53.866) -> (-66, -54.7321)
  line L1810 (-66.5, -38.866) -> (-66, -39.7321)
  line L1811 (-69, -48.7321) -> (-68, -48.7321)
  line L1812 (-54, -54.7321) -> (-53, -54.7321)
  line L1813 (-66, -36.7321) -> (-65, -36.7321)
  line L1814 (-67.5, -35.866) -> (-68, -35)
  line L1815 (-68, -47) -> (-69, -47)
  line L1816 (-54, -51.7321) -> (-53, -51.7321)
  line L1817 (-57.5, -56.866) -> (-57, -57.7321)
  line L1818 (-53, -53) -> (-54, -53)
  line L1819 (-66, -44) -> (-66.5, -44.866)
  line L1820 (-57.5, -53.866) -> (-57, -54.7321)
  line L1821 (-57.5, -50.866) -> (-57, -51.7321)
  line L1822 (-66, -47) -> (-66.5, -47.866)
  line L1823 (-55.5, -56.866) -> (-56, -56)
  line L1824 (-69.5, -47.866) -> (-69, -48.7321)
  line L1825 (-67.5, -41.866) -> (-68, -41)
  line L1826 (-56, -51.7321) -> (-55.5, -50.866)
  line L1827 (-56, -57.7321) -> (-55.5, -56.866)
  line L1828 (-56, -53) -> (-57, -53)
  line L1829 (-54, -57.7321) -> (-53, -57.7321)
  line L1830 (-57, -54.7321) -> (-56, -54.7321)
  line L1831 (-54, -50) -> (-54.5, -50.866)
  line L1832 (-65, -47) -> (-66, -47)
  line L1833 (-66.5, -35.866) -> (-66, -36.7321)
  line L1834 (-57, -51.7321) -> (-56, -51.7321)
  line L1835 (-56, -56) -> (-57, -56)
  line L1836 (-68, -36.7321) -> (-67.5, -35.866)
  line L1837 (-65, -41) -> (-66, -41)
  line L1838 (-54.5, -53.866) -> (-54, -54.7321)
  line L1839 (-68, -44) -> (-69, -44)
  line L1840 (-65, -48.7321) -> (-64.5, -47.866)
  line L1841 (-67.5, -47.866) -> (-68, -47)
  line L1842 (-64.5, -47.866) -> (-65, -47)
  line L1843 (-69.5, -41.866) -> (-69, -42.7321)
  line L1844 (-55.5, -53.866) -> (-56, -53)
  line L1845 (-66, -48.7321) -> (-65, -48.7321)
  line L1846 (-66, -41) -> (-66.5, -41.866)
  line L1847 (-69, -44) -> (-69.5, -44.866)
  line L1848 (-57, -53) -> (-57.5, -53.866)
  line L1849 (-65, -45.7321) -> (-64.5, -44.866)
  line L1850 (-68, -41) -> (-69, -41)
  line L1851 (-54, -56) -> (-54.5, -56.866)
  line L1852 (-56, -50) -> (-57, -50)
  line L1853 (-69, -41) -> (-69.5, -41.866)
  line L1854 (-25.5, -53.866) -> (-26, -53)
  line L1855 (-24, -53) -> (-24.5, -53.866)
  line L1856 (-30, -48.7321) -> (-29, -48.7321)
  line L1857 (-25.5, -56.866) -> (-26, -56)
  line L1858 (-27, -50) -> (-27.5, -50.866)
  line L1859 (-25.5, -50.866) -> (-26, -50)
  line L1860 (-32, -42.7321) -> (-31.5, -41.866)
  line L1861 (-32, -44) -> (-33, -44)
  line L1862 (-32, -45.7321) -> (-31.5, -44.866)
  line L1863 (-23, -53) -> (-24, -53)
  line L1864 (-26, -53) -> (-27, -53)
  line L1865 (-33, -47) -> (-33.5, -47.866)
  line L1866 (-24, -51.7321) -> (-23, -51.7321)
  line L1867 (-26, -54.7321) -> (-25.5, -53.866)
  line L1868 (-27.5, -53.866) -> (-27, -54.7321)
  line L1869 (-24.5, -56.866) -> (-24, -57.7321)
  line L1870 (-33, -42.7321) -> (-32, -42.7321)
  line L1871 (-30, -41) -> (-30.5, -41.866)
  line L1872 (-30, -44) -> (-30.5, -44.866)
  line L1873 (-27.5, -56.866) -> (-27, -57.7321)
  line L1874 (-32, -48.7321) -> (-31.5, -47.866)
  line L1875 (-27, -56) -> (-27.5, -56.866)
  line L1876 (-27.5, -50.866) -> (-27, -51.7321)
  line L1877 (-27, -57.7321) -> (-26, -57.7321)
  line L1878 (-29, -44) -> (-30, -44)
  line L1879 (-23, -50) -> (-24, -50)
  line L1880 (-27, -53) -> (-27.5, -53.866)
  line L1881 (-24.5, -53.866) -> (-24, -54.7321)
  line L1882 (-33, -48.7321) -> (-32, -48.7321)
  line L1883 (-28.5, -41.866) -> (-29, -41)
  line L1884 (-24, -57.7321) -> (-23, -57.7321)
  line L1885 (-24.5, -50.866) -> (-24, -51.7321)
  line L1886 (-23, -56) -> (-24, -56)
  line L1887 (-24, -56) -> (-24.5, -56.866)
  line L1888 (-24, -50) -> (-24.5, -50.866)
  line L1889 (-28.5, -44.866) -> (-29, -44)
  line L1890 (-29, -48.7321) -> (-28.5, -47.866)
  line L1891 (-29, -41) -> (-30, -41)
  line L1892 (-24, -54.7321) -> (-23, -54.7321)
  line L1893 (-26, -57.7321) -> (-25.5, -56.866)
  line L1894 (-27, -51.7321) -> (-26, -51.7321)
  line L1895 (-31.5, -44.866) -> (-32, -44)
  line L1896 (-32, -41) -> (-33, -41)
  line L1897 (-27, -54.7321) -> (-26, -54.7321)
  line L1898 (-48, -36.7321) -> (-47, -36.7321)
  line L1899 (-41, -36.7321) -> (-40.5, -35.866)
  line L1900 (-45.5, -35.866) -> (-45, -36.7321)
  line L1901 (-42, -39.7321) -> (-41, -39.7321)
  line L1902 (-47, -36.7321) -> (-46.5, -35.866)
  line L1903 (-30.5, -44.866) -> (-30, -45.7321)
  line L1904 (-44, -39.7321) -> (-43.5, -38.866)
  line L1905 (-46.5, -38.866) -> (-47, -38)
  line L1906 (-48, -38) -> (-48.5, -38.866)
  line L1907 (-48.5, -35.866) -> (-48, -36.7321)
  line L1908 (-30, -45.7321) -> (-29, -45.7321)
  line L1909 (-29, -42.7321) -> (-28.5, -41.866)
  line L1910 (-26, -50) -> (-27, -50)
  line L1911 (-33, -41) -> (-33.5, -41.866)
  line L1912 (-26, -51.7321) -> (-25.5, -50.866)
  line L1913 (-33.5, -47.866) -> (-33, -48.7321)
  line L1914 (-32, -57.7321) -> (-31.5, -56.866)
  line L1915 (-47, -35) -> (-48, -35)
  line L1916 (-26, -56) -> (-27, -56)
  line L1917 (-46.5, -35.866) -> (-47, -35)
  line L1918 (-47, -38) -> (-48, -38)
  line L1919 (-40.5, -35.866) -> (-41, -35)
  line L1920 (-48, -35) -> (-48.5, -35.866)
  line L1921 (-45, -39.7321) -> (-44, -39.7321)
  line L1922 (-42, -36.7321) -> (-41, -36.7321)
  line L1923 (-33.5, -44.866) -> (-33, -45.7321)
  line L1924 (-62, -72.7321) -> (-61.5, -71.866)
  line L1925 (-60.5, -74.866) -> (-60, -75.7321)
  line L1926 (-62, -74) -> (-63, -74)
  line L1927 (-59, -75.7321) -> (-58.5, -74.866)
  line L1928 (-65, -66.7321) -> (-64.5, -65.866)
  line L1929 (-67.5, -62.866) -> (-68, -62)
  line L1930 (-66.5, -74.866) -> (-66, -75.7321)
  line L1931 (-68, -68) -> (-69, -68)
  line L1932 (-67.5, -71.866) -> (-68, -71)
  line L1933 (-69, -72.7321) -> (-68, -72.7321)
  line L1934 (-66, -69.7321) -> (-65, -69.7321)
  line L1935 (-69, -63.7321) -> (-68, -63.7321)
  line L1936 (-68, -65) -> (-69, -65)
  line L1937 (-69.5, -71.866) -> (-69, -72.7321)
  line L1938 (-69.5, -74.866) -> (-69, -75.7321)
  line L1939 (-69, -62) -> (-69.5, -62.866)
  line L1940 (-66, -74) -> (-66.5, -74.866)
  line L1941 (-65, -72.7321) -> (-64.5, -71.866)
  line L1942 (-69, -69.7321) -> (-68, -69.7321)
  line L1943 (-64.5, -74.866) -> (-65, -74)
  line L1944 (-68, -62) -> (-69, -62)
  line L1945 (-69, -66.7321) -> (-68, -66.7321)
  line L1946 (-64.5, -65.866) -> (-65, -65)
  line L1947 (-66.5, -65.866) -> (-66, -66.7321)
  line L1948 (-65, -65) -> (-66, -65)
  line L1949 (-65, -68) -> (-66, -68)
  line L1950 (-67.5, -68.866) -> (-68, -68)
  line L1951 (-66, -65) -> (-66.5, -65.866)
  line L1952 (-68, -63.7321) -> (-67.5, -62.866)
  line L1953 (-66, -62) -> (-66.5, -62.866)
  line L1954 (-66, -68) -> (-66.5, -68.866)
  line L1955 (-69, -68) -> (-69.5, -68.866)
  line L1956 (-65, -63.7321) -> (-64.5, -62.866)
  line L1957 (-66.5, -62.866) -> (-66, -63.7321)
  line L1958 (-66, -66.7321) -> (-65, -66.7321)
  line L1959 (-65, -62) -> (-66, -62)
  line L1960 (-68, -66.7321) -> (-67.5, -65.866)
  line L1961 (-69.5, -62.866) -> (-69, -63.7321)
  line L1962 (-67.5, -65.866) -> (-68, -65)
  line L1963 (-66, -63.7321) -> (-65, -63.7321)
  line L1964 (-64.5, -68.866) -> (-65, -68)
  line L1965 (-69.5, -65.866) -> (-69, -66.7321)
  line L1966 (-39, -75.7321) -> (-38, -75.7321)
  line L1967 (-55.5, -71.866) -> (-56, -71)
  line L1968 (-36, -71) -> (-36.5, -71.866)
  line L1969 (-56, -68) -> (-57, -68)
  line L1970 (-57, -68) -> (-57.5, -68.866)
  line L1971 (-57.5, -74.866) -> (-57, -75.7321)
  line L1972 (-56, -75.7321) -> (-55.5, -74.866)
  line L1973 (-54.5, -71.866) -> (-54, -72.7321)
  line L1974 (-54.5, -68.866) -> (-54, -69.7321)
  line L1975 (-54.5, -74.866) -> (-54, -75.7321)
  line L1976 (-55.5, -68.866) -> (-56, -68)
  line L1977 (-38, -75.7321) -> (-37.5, -74.866)
  line L1978 (-55.5, -74.866) -> (-56, -74)
  line L1979 (-57, -75.7321) -> (-56, -75.7321)
  line L1980 (-56, -72.7321) -> (-55.5, -71.866)
  line L1981 (-54, -74) -> (-54.5, -74.866)
  line L1982 (-57, -69.7321) -> (-56, -69.7321)
  line L1983 (-57, -74) -> (-57.5, -74.866)
  line L1984 (-56, -71) -> (-57, -71)
  line L1985 (-56, -69.7321) -> (-55.5, -68.866)
  line L1986 (-57.5, -71.866) -> (-57, -72.7321)
  line L1987 (-57.5, -68.866) -> (-57, -69.7321)
  line L1988 (-38, -74) -> (-39, -74)
  line L1989 (-37.5, -74.866) -> (-38, -74)
  line L1990 (-36, -69.7321) -> (-35, -69.7321)
  line L1991 (-54, -71) -> (-54.5, -71.866)
  line L1992 (-37.5, -71.866) -> (-38, -71)
  line L1993 (-65, -60.7321) -> (-64.5, -59.866)
  line L1994 (-69, -60.7321) -> (-68, -60.7321)
  line L1995 (-57, -71) -> (-57.5, -71.866)
  line L1996 (-56, -74) -> (-57, -74)
  line L1997 (-69, -65) -> (-69.5, -65.866)
  line L1998 (-66, -60.7321) -> (-65, -60.7321)
  line L1999 (-54, -68) -> (-54.5, -68.866)
  line L2000 (-64.5, -59.866) -> (-65, -59)
  line L2001 (-64.5, -62.866) -> (-65, -62)
  line L2002 (-57, -72.7321) -> (-56, -72.7321)
  line L2003 (-65, -59) -> (-66, -59)
  line L2004 (-67.5, -59.866) -> (-68, -59)
  line L2005 (-66, -59) -> (-66.5, -59.866)
  line L2006 (-68, -60.7321) -> (-67.5, -59.866)
  line L2007 (-69.5, -59.866) -> (-69, -60.7321)
  line L2008 (-66.5, -59.866) -> (-66, -60.7321)
  line L2009 (-69, -59) -> (-69.5, -59.866)
  line L2010 (-68, -59) -> (-69, -59)
  line L2011 (-69, -75.7321) -> (-68, -75.7321)
  line L2012 (-65, -71) -> (-66, -71)
  line L2013 (-69, -74) -> (-69.5, -74.866)
  line L2014 (-68, -69.7321) -> (-67.5, -68.866)
  line L2015 (-66.5, -71.866) -> (-66, -72.7321)
  line L2016 (-62, -60.7321) -> (-61.5, -59.866)
  line L2017 (-63, -60.7321) -> (-62, -60.7321)
  line L2018 (-68, -72.7321) -> (-67.5, -71.866)
  line L2019 (-67.5, -74.866) -> (-68, -74)
  line L2020 (-66, -71) -> (-66.5, -71.866)
  line L2021 (-66, -75.7321) -> (-65, -75.7321)
  line L2022 (-65, -69.7321) -> (-64.5, -68.866)
  line L2023 (-64.5, -71.866) -> (-65, -71)
  line L2024 (-65, -74) -> (-66, -74)
  line L2025 (-63, -59) -> (-63.5, -59.866)
  line L2026 (-61.5, -59.866) -> (-62, -59)
  line L2027 (-68, -71) -> (-69, -71)
  line L2028 (-58.5, -59.866) -> (-59, -59)
  line L2029 (-60.5, -59.866) -> (-60, -60.7321)
  line L2030 (-62, -59) -> (-63, -59)
  line L2031 (-68, -75.7321) -> (-67.5, -74.866)
  line L2032 (-68, -74) -> (-69, -74)
  line L2033 (-59, -59) -> (-60, -59)
  line L2034 (-65, -75.7321) -> (-64.5, -74.866)
  line L2035 (-60, -60.7321) -> (-59, -60.7321)
  line L2036 (-69.5, -68.866) -> (-69, -69.7321)
  line L2037 (-66, -72.7321) -> (-65, -72.7321)
  line L2038 (-66.5, -68.866) -> (-66, -69.7321)
  line L2039 (-69, -71) -> (-69.5, -71.866)
  line L2040 (-14, -65) -> (-15, -65)
  line L2041 (-15, -60.7321) -> (-14, -60.7321)
  line L2042 (-10.5, -68.866) -> (-11, -68)
  line L2043 (-12.5, -59.866) -> (-12, -60.7321)
  line L2044 (-10.5, -65.866) -> (-11, -65)
  line L2045 (-14, -60.7321) -> (-13.5, -59.866)
  line L2046 (-10.5, -59.866) -> (-11, -59)
  line L2047 (-12, -59) -> (-12.5, -59.866)
  line L2048 (-13.5, -59.866) -> (-14, -59)
  line L2049 (-12, -66.7321) -> (-11, -66.7321)
  line L2050 (-14, -63.7321) -> (-13.5, -62.866)
  line L2051 (-13.5, -68.866) -> (-14, -68)
  line L2052 (-15, -63.7321) -> (-14, -63.7321)
  line L2053 (-15, -69.7321) -> (-14, -69.7321)
  line L2054 (-12, -60.7321) -> (-11, -60.7321)
  line L2055 (-13.5, -65.866) -> (-14, -65)
  line L2056 (-13.5, -62.866) -> (-14, -62)
  line L2057 (-13.5, -74.866) -> (-14, -74)
  line L2058 (-15, -72.7321) -> (-14, -72.7321)
  line L2059 (-14, -62) -> (-15, -62)
  line L2060 (-15, -66.7321) -> (-14, -66.7321)
  line L2061 (-15, -75.7321) -> (-14, -75.7321)
  line L2062 (-14, -59) -> (-15, -59)
  line L2063 (-14, -74) -> (-15, -74)
  line L2064 (-14, -71) -> (-15, -71)
  line L2065 (-14, -68) -> (-15, -68)
  line L2066 (-11, -60.7321) -> (-10.5, -59.866)
  line L2067 (-11, -71) -> (-12, -71)
  line L2068 (-11, -59) -> (-12, -59)
  line L2069 (-13.5, -71.866) -> (-14, -71)
  line L2070 (-11, -74) -> (-12, -74)
  line L2071 (-12.5, -71.866) -> (-12, -72.7321)
  line L2072 (-12, -63.7321) -> (-11, -63.7321)
  line L2073 (-12, -65) -> (-12.5, -65.866)
  line L2074 (-14, -69.7321) -> (-13.5, -68.866)
  line L2075 (-11, -68) -> (-12, -68)
  line L2076 (-12, -75.7321) -> (-11, -75.7321)
  line L2077 (-12.5, -62.866) -> (-12, -63.7321)
  line L2078 (-11, -62) -> (-12, -62)
  line L2079 (-11, -66.7321) -> (-10.5, -65.866)
  line L2080 (-10.5, -74.866) -> (-11, -74)
  line L2081 (-14, -66.7321) -> (-13.5, -65.866)
  line L2082 (-11, -65) -> (-12, -65)
  line L2083 (-12, -69.7321) -> (-11, -69.7321)
  line L2084 (-12, -71) -> (-12.5, -71.866)
  line L2085 (-12, -72.7321) -> (-11, -72.7321)
  line L2086 (-14, -75.7321) -> (-13.5, -74.866)
  line L2087 (-10.5, -62.866) -> (-11, -62)
  line L2088 (-11, -69.7321) -> (-10.5, -68.866)
  line L2089 (-12.5, -74.866) -> (-12, -75.7321)
  line L2090 (-12.5, -65.866) -> (-12, -66.7321)
  line L2091 (-12, -68) -> (-12.5, -68.866)
  line L2092 (-14, -72.7321) -> (-13.5, -71.866)
  line L2093 (-12, -74) -> (-12.5, -74.866)
  line L2094 (-11, -72.7321) -> (-10.5, -71.866)
  line L2095 (-12, -62) -> (-12.5, -62.866)
  line L2096 (-11, -75.7321) -> (-10.5, -74.866)
  line L2097 (-12.5, -68.866) -> (-12, -69.7321)
  line L2098 (-11, -63.7321) -> (-10.5, -62.866)
  line L2099 (-10.5, -71.866) -> (-11, -71)
  line L2100 (-47, -71) -> (-48, -71)
  line L2101 (-29, -63.7321) -> (-28.5, -62.866)
  line L2102 (-46.5, -71.866) -> (-47, -71)
  line L2103 (-45, -74) -> (-45.5, -74.866)
  line L2104 (-30, -63.7321) -> (-29, -63.7321)
  line L2105 (-48, -69.7321) -> (-47, -69.7321)
  line L2106 (-33.5, -68.866) -> (-33, -69.7321)
  line L2107 (-48.5, -74.866) -> (-48, -75.7321)
  line L2108 (-33.5, -62.866) -> (-33, -63.7321)
  line L2109 (-31.5, -62.866) -> (-32, -62)
  line L2110 (-48, -68) -> (-48.5, -68.866)
  line L2111 (-45, -71) -> (-45.5, -71.866)
  line L2112 (-45.5, -68.866) -> (-45, -69.7321)
  line L2113 (-32, -62) -> (-33, -62)
  line L2114 (-30.5, -65.866) -> (-30, -66.7321)
  line L2115 (-30, -62) -> (-30.5, -62.866)
  line L2116 (-29, -72.7321) -> (-28.5, -71.866)
  line L2117 (-33, -69.7321) -> (-32, -69.7321)